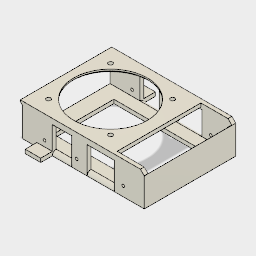
hard-drive-enclosure-v6 (Autodesk Fusion 360 design; units mm, degrees)
Autodesk Fusion 360 part; units mm, degrees
sketch "Sketch1" plane through (0, 0, 0) normal (0, 1, 0) x (1, 0, 0)
  line L0 (68.6494, -55) -> (-78.3404, -55)
  line L1 (-78.3404, -55) -> (-78.3404, 53)
  line L2 (-78.3404, 53) -> (68.6494, 53)
  line L3 (68.6494, 53) -> (68.6494, -55)
  line L4 (78.6494, 58) -> (-78.6124, 58)
  line L5 (-78.6124, 58) -> (-78.6124, -60)
  line L6 (-78.6124, -60) -> (78.6494, -60)
  line L7 (78.6494, -60) -> (78.6494, 58)
  dimension "d1" = 146.9898
  dimension "d2" = 108
  dimension "d3" = 5
  dimension "d4" = 5
  dimension "d5" = 10
  measures "d1" distance of L1 L3
  measures "d2" distance of L0 L2
  measures "d3" distance of L2 L4
  measures "d4" distance of L0 L6
  measures "d5" distance of L3 L7
extrude "Extrude1" add sketch "Sketch1" along normal blind 5 contours L0 L1 L2 L3 | L4 L5 L6 L7
sketch "Sketch2" plane through (0, 5, 0) normal (0, 1, 0) x (-1, 0, 0)
  line L0 (-78.6494, 60) -> (-78.6494, -58)
  line L1 (-78.6494, -58) -> (78.6124, -58)
  line L2 (78.6124, -58) -> (78.6124, 60)
  line L3 (78.6124, 60) -> (-78.6494, 60)
  line L4 (78.6124, -53) -> (-68.6494, -53)
  line L5 (-68.6494, -53) -> (-68.6494, 55)
  line L6 (-68.6494, 55) -> (78.6124, 55)
  line L7 (78.6124, 55) -> (78.6124, -53)
  line L8 (78.6124, -58) -> (-78.6494, -58)
  line L9 (-78.6494, -58) -> (-78.6494, 60)
  line L10 (-78.6494, 60) -> (78.6124, 60)
  line L11 (78.6124, 60) -> (78.6124, -58)
  dimension "d8" = 5
  dimension "d9" = 5
  dimension "d10" = 10
  measures "d8" distance of L1 L4
  measures "d9" distance of L3 L6
  measures "d10" distance of L0 L5
extrude "Extrude2" add sketch "Sketch2" along normal blind 27 contours L0 L1 L2 L3 L4 L5 L6 L8 L9 L10 L11
sketch "Sketch3" plane through (0, 32, 0) normal (0, 1, 0) x (-1, 0, 0)
  line L0 (78.6124, -53) -> (-68.6494, -53)
  line L1 (-68.6494, -53) -> (-68.6494, 55)
  line L2 (-68.6494, 55) -> (78.6124, 55)
  line L3 (78.6124, 55) -> (78.6124, 60)
  line L4 (78.6124, 60) -> (-78.6494, 60)
  line L5 (-78.6494, 60) -> (-78.6494, -58)
  line L6 (-78.6494, -58) -> (78.6124, -58)
  line L7 (78.6124, -58) -> (78.6124, -53)
  line L8 (56.3506, -58) -> (26.3506, -58)
  line L9 (26.3506, -58) -> (26.3506, 60)
  line L10 (26.3506, 60) -> (56.3506, 60)
  line L11 (56.3506, 60) -> (56.3506, -58)
  line L12 (-43.6494, 60) -> (-13.6494, 60)
  line L13 (-13.6494, 60) -> (-13.6494, -58)
  line L14 (-13.6494, -58) -> (-43.6494, -58)
  line L15 (-43.6494, -58) -> (-43.6494, 60)
  dimension "d13" = 112
  dimension "d14" = 30
  dimension "d15" = 30
  dimension "d16" = 40
  dimension "d17" = 25
  measures "d14" distance of L13 L15
  measures "d15" distance of L9 L11
  measures "d16" distance of L9 L13
  measures "d17" distance of L1 L15
extrude "Extrude3" add sketch "Sketch3" along normal blind 5 contours L0 L6 L7 L11 | L0 L6 L8 L9 L11 | L0 L6 L9 L13 | L0 L2 L9 L13 | L2 L3 L4 L11 | L2 L4 L9 L10 L11 | L0 L6 L13 L14 L15 | L2 L4 L9 L13 | L0 L1 L2 L4 L5 L6 L15 | L2 L4 L12 L13 L15
sketch "Sketch4" plane through (0, 0, 0) normal (0, -1, 0) x (1, 0, 0)
  line L0 (78.6494, -58) -> (78.6494, 60)
  line L1 (78.6494, 60) -> (-78.6124, 60)
  line L2 (-78.6124, 60) -> (-78.6124, -58)
  line L3 (-78.6124, -58) -> (78.6494, -58)
  line L4 (-60, 75) -> (-40, 75)
  line L5 (-40, 75) -> (-40, -73)
  line L6 (-40, -73) -> (-60, -73)
  line L7 (-60, -73) -> (-60, 75)
  line L8 (50, -73) -> (30, -73)
  line L9 (30, -73) -> (30, 75)
  line L10 (30, 75) -> (50, 75)
  line L11 (50, 75) -> (50, -73)
  dimension "d20" = 15
  dimension "d21" = 15
  dimension "d22" = 15
  dimension "d23" = 15
  measures "d20" distance of L1 L10
  measures "d21" distance of L3 L8
  measures "d22" distance of L3 L6
  measures "d23" distance of L1 L4
extrude "Extrude4" add sketch "Sketch4" against normal blind 5 contours L3 L8 L9 L11 | L1 L9 L10 L11 | L3 L5 L6 L7 | L1 L4 L5 L7
sketch "Sketch5" plane through (0, 0, 60) normal (0, 0, 1) x (1, 0, 0)
  line L0 (50, 5) -> (50, 0)
  line L1 (50, 0) -> (78.6494, 0)
  line L2 (78.6494, 0) -> (78.6494, 37)
  line L3 (78.6494, 37) -> (-78.6124, 37)
  line L4 (-78.6124, 37) -> (-78.6124, 0)
  line L5 (-78.6124, 0) -> (-60, 0)
  line L6 (-60, 0) -> (-60, 5)
  line L7 (-60, 5) -> (-40, 5)
  line L8 (-40, 5) -> (-40, 0)
  line L9 (-40, 0) -> (30, 0)
  line L10 (30, 0) -> (30, 5)
  line L11 (30, 5) -> (50, 5)
  circle A0 centre (-50.1136, 12.35) radius 1.7525
  circle A1 centre (-8.5084, 12.35) radius 1.7525
  circle A2 centre (51.4864, 12.35) radius 1.7525
  dimension "d26" = 12.35
  dimension "d27" = 12.35
  dimension "d28" = 12.35
  dimension "d29" = 3.505
  dimension "d30" = 3.505
  dimension "d31" = 3.505
  dimension "d32" = 28.4988
  dimension "d33" = 41.6052
  dimension "d34" = 101.6
  measures "d26" distance of L1 A2.centre
  measures "d27" distance of L9 A1.centre
  measures "d28" distance of L9 A0.centre
  measures "d29" diameter of A2
  measures "d30" diameter of A1
  measures "d31" diameter of A0
  measures "d32" distance of L4 A0.centre
  measures "d33" distance of A0.centre A1.centre
  measures "d34" distance of A0.centre A2.centre
extrude "Extrude5" cut sketch "Sketch5" against normal blind 170 contours A0 | A1 | A2
delete_face "DeleteFace1" 1 faces at (43.3333, 5, 65)
delete_face "DeleteFace2" 1 faces at (43.3333, 5, -68)
sketch "Sketch6" plane through (0, 0, 0) normal (0, -1, 0) x (1, 0, 0)
  line L0 (-60, -58) -> (-60, -73)
  line L1 (-60, -73) -> (-40, -73)
  line L2 (-40, -73) -> (-40, -58)
  line L3 (-40, -58) -> (78.6494, -58)
  line L4 (78.6494, -58) -> (78.6494, 60)
  line L5 (78.6494, 60) -> (-40, 60)
  line L6 (-40, 60) -> (-40, 75)
  line L7 (-40, 75) -> (-60, 75)
  line L8 (-60, 75) -> (-60, 60)
  line L9 (-60, 60) -> (-78.6124, 60)
  line L10 (-78.6124, 60) -> (-78.6124, -58)
  line L11 (-78.6124, -58) -> (-60, -58)
  line L12 (-58.6124, 40) -> (58.6494, 40)
  line L13 (58.6494, 40) -> (58.6494, -38)
  line L14 (58.6494, -38) -> (-58.6124, -38)
  line L15 (-58.6124, -38) -> (-58.6124, 40)
  dimension "d37" = 20
  dimension "d38" = 20
  dimension "d39" = 20
  dimension "d40" = 20
  measures "d37" distance of L5 L12
  measures "d38" distance of L3 L14
  measures "d39" distance of L4 L13
  measures "d40" distance of L10 L15
extrude "Extrude6" cut sketch "Sketch6" against normal blind 10 contours L12 L13 L14 L15
sketch "Sketch7" plane through (0, 37, 0) normal (0, 1, 0) x (-1, 0, 0)
  line L0 (-13.6494, -53) -> (-68.6494, -53)
  line L1 (-68.6494, -53) -> (-68.6494, 55)
  line L2 (-68.6494, 55) -> (-13.6494, 55)
  line L3 (-13.6494, 55) -> (-13.6494, -53)
  line L4 (-78.6494, -58) -> (78.6124, -58)
  line L5 (78.6124, -58) -> (78.6124, -53)
  line L6 (78.6124, -53) -> (26.3506, -53)
  line L7 (26.3506, -53) -> (26.3506, 55)
  line L8 (26.3506, 55) -> (78.6124, 55)
  line L9 (78.6124, 55) -> (78.6124, 60)
  line L10 (78.6124, 60) -> (-78.6494, 60)
  line L11 (-78.6494, 60) -> (-78.6494, -58)
  line L12 (26.3506, -53) -> (-13.6494, -53)
  line L13 (-13.6494, -53) -> (-13.6494, 55)
  line L14 (-13.6494, 55) -> (26.3506, 55)
  line L15 (26.3506, 55) -> (26.3506, -53)
extrude "Extrude7" cut sketch "Sketch7" against normal blind 10 contours L3 L7 L12 L13 L14 L15
sketch "Sketch8" plane through (0, 37, 0) normal (0, 1, 0) x (-1, 0, 0)
  line L0 (78.6124, -53) -> (-68.6494, -53)
  line L1 (-68.6494, -53) -> (-68.6494, 55)
  line L2 (-68.6494, 55) -> (78.6124, 55)
  line L3 (78.6124, 55) -> (78.6124, 60)
  line L4 (78.6124, 60) -> (-78.6494, 60)
  line L5 (-78.6494, 60) -> (-78.6494, -58)
  line L6 (-78.6494, -58) -> (78.6124, -58)
  line L7 (78.6124, -58) -> (78.6124, -53)
  line L8 (81.3506, -58) -> (-38.6494, -58)
  line L9 (-38.6494, -58) -> (-38.6494, 60)
  line L10 (-38.6494, 60) -> (81.3506, 60)
  line L11 (81.3506, 60) -> (81.3506, -58)
  dimension "d45" = 120
  dimension "d46" = 30
  measures "d45" distance of L9 L11
  measures "d46" distance of L1 L9
extrude "Extrude8" add sketch "Sketch8" along normal blind 5 contours L0 L6 L7 L8 L9 | L0 L2 L3 L7 L8 L9 L10 L11 | L2 L3 L4 L9 L10
move_face "OffsetFaces1" offset 2 1 faces at (-39.5252, 37, 19)
sketch "Sketch9" plane through (0, 42, 0) normal (0, 1, 0) x (-1, 0, 0)
  line L0 (81.3506, 60) -> (-38.6494, 60)
  line L1 (-38.6494, 60) -> (-38.6494, -58)
  line L2 (-38.6494, -58) -> (81.3506, -58)
  line L3 (81.3506, -58) -> (81.3506, 60)
  line L4 (71.3506, -46.5) -> (-23.6494, -46.5)
  line L5 (-23.6494, -46.5) -> (-23.6494, 48.5)
  line L6 (-23.6494, 48.5) -> (71.3506, 48.5)
  line L7 (71.3506, 48.5) -> (71.3506, -46.5)
  circle A0 centre (23.8506, 1) radius 47.5
  circle A1 centre (63.8506, -39) radius 2.8
  line L8 (58.6124, -38) -> (58.6124, 40)
  line L9 (-58.6494, -38) -> (58.6124, -38)
  circle A2 centre (-16.1494, 41) radius 2.8
  circle A3 centre (63.8506, 41) radius 2.8
  circle A4 centre (-16.1494, -39) radius 2.8
  dimension "d50" = 95
  dimension "d51" = 95
  dimension "d52" = 11.5
  dimension "d53" = 8
  dimension "d54" = 15
  dimension "d55" = 2.5
  dimension "d56" = 5.6
  dimension "d57" = 5.6
  dimension "d58" = 5.6
  dimension "d60" = 7.5
  dimension "d61" = 7.5
  dimension "d64" = 7.5
  dimension "d65" = 7.5
  dimension "d66" = 7.5
  dimension "d67" = 7.5
  dimension "d79" = 2.5
  dimension "d81" = 5.6
  dimension "d82" = 7.5
  dimension "d83" = 7.5
  measures "d50" distance of L5 L7
  measures "d51" distance of L4 L6
  measures "d52" distance of L0 L6
  measures "d54" distance of L1 L5
  measures "d56" diameter of A3
  measures "d57" diameter of A1
  measures "d58" diameter of A2
  measures "d60" distance of L4 A1.centre
  measures "d61" distance of L7 A1.centre
  measures "d64" distance of L5 A2.centre
  measures "d65" distance of L6 A2.centre
  measures "d66" distance of L6 A3.centre
  measures "d67" distance of L7 A3.centre
  measures "d81" diameter of A4
  measures "d82" distance of L5 A4.centre
  measures "d83" distance of L4 A4.centre
extrude "Extrude9" cut sketch "Sketch9" against normal blind 20 contours A0 L9 | A0 L8 | A0 L8 L9 | L9 A4 | L9 A4 | A1 | A2 | A3 picked at (37.1903, -12.7965)
sketch "Sketch10" plane through (0, 0, 60) normal (0, 0, 1) x (1, 0, 0)
  circle A0 centre (51.4864, 12.35) radius 1.7525
  circle A1 centre (-8.5084, 12.35) radius 1.7525
  circle A2 centre (-50.1136, 12.35) radius 1.7525
  line L0 (-78.6124, 35) -> (-78.6124, 0)
  line L1 (-78.6124, 0) -> (-60, 0)
  line L2 (-60, 0) -> (-60, 5)
  line L3 (-60, 5) -> (-40, 5)
  line L4 (-40, 5) -> (-40, 0)
  line L5 (-40, 0) -> (78.6494, 0)
  line L6 (78.6494, 0) -> (78.6494, 37)
  line L7 (78.6494, 37) -> (38.6494, 37)
  line L8 (38.6494, 37) -> (38.6494, 42)
  line L9 (38.6494, 42) -> (-81.3506, 42)
  line L10 (-81.3506, 42) -> (-81.3506, 35)
  line L11 (-81.3506, 35) -> (-78.6124, 35)
  line L12 (-40, 0) -> (-15, 0)
  line L13 (-15, 0) -> (-15, 35)
  line L14 (-15, 35) -> (-40, 35)
  line L15 (-40, 35) -> (-40, 0)
  line L16 (-78.6124, 35) -> (38.6494, 35)
  line L17 (5, 35) -> (40, 35)
  line L18 (40, 35) -> (40, 5)
  line L19 (40, 5) -> (5, 5)
  line L20 (5, 5) -> (5, 35)
  line L21 (-40, 35) -> (-15, 35)
  line L22 (-15, 35) -> (-15, 5)
  line L23 (-15, 5) -> (-40, 5)
  line L24 (-40, 5) -> (-40, 35)
  dimension "d70" = 25
  dimension "d71" = 35
  dimension "d72" = 30
  dimension "d73" = 20
  dimension "d76" = 35
  measures "d70" distance of L13 L15
  measures "d71" distance of L18 L20
  measures "d72" distance of L17.start L19.end
  measures "d73" distance of L13 L20
  measures "d76" distance of L12 L14
extrude "Extrude11" cut sketch "Sketch10" against normal blind 175 contours L13 L14 L15 L16 L21 L22 L23 L24 | L16 L17 L18 L19 L20
sketch "Sketch11" plane through (0, 0, 0) normal (0, -1, 0) x (1, 0, 0)
  line L0 (58.6494, 40) -> (58.6494, -38)
  line L1 (58.6494, -38) -> (-58.6124, -38)
  line L2 (-58.6124, -38) -> (-58.6124, 40)
  line L3 (-58.6124, 40) -> (58.6494, 40)
  line L4 (-60, -58) -> (-60, -73)
  line L5 (-60, -73) -> (-40, -73)
  line L6 (-40, -73) -> (-40, -58)
  line L7 (-40, -58) -> (78.6494, -58)
  line L8 (78.6494, -58) -> (78.6494, 60)
  line L9 (78.6494, 60) -> (-40, 60)
  line L10 (-40, 60) -> (-40, 75)
  line L11 (-40, 75) -> (-60, 75)
  line L12 (-60, 75) -> (-60, 60)
  line L13 (-60, 60) -> (-78.6124, 60)
  line L14 (-78.6124, 60) -> (-78.6124, -58)
  line L15 (-78.6124, -58) -> (-60, -58)
chamfer "Chamfer1" distance 5 angle 45 1 edges at (20.4349, 35, -16.1767)
fillet "Fillet1" radius 22.5 1 edges at (68.6494, 37, 1)
fillet "Fillet2" radius 5 4 edges at (-27.5, 5, -58) (22.5, 5, -58) (22.5, 5, 60) (-27.5, 5, 60)
sketch "Sketch12" plane through (0, 37, 0) normal (0, 1, 0) x (-1, 0, 0)
  line L0 (-78.6494, 55) -> (-38.6494, 55)
  line L1 (-38.6494, 55) -> (-38.6494, 60)
  line L2 (-38.6494, 60) -> (-78.6494, 60)
  line L3 (-78.6494, 60) -> (-78.6494, 55)
  line L4 (-38.6494, 55) -> (-78.6494, 55)
  line L5 (-78.6494, 55) -> (-78.6494, 60)
  line L6 (-78.6494, 60) -> (-38.6494, 60)
  line L7 (-38.6494, 60) -> (-38.6494, 55)
  line L8 (-38.6494, -58) -> (-78.6494, -58)
  line L9 (-78.6494, -58) -> (-78.6494, -53)
  line L10 (-78.6494, -53) -> (-38.6494, -53)
  line L11 (-38.6494, -53) -> (-38.6494, -58)
  point P0 (-38.6494, -58)
  point P1 (-78.6494, -53)
extrude "Extrude12" add sketch "Sketch12" along normal blind 5
chamfer "Chamfer2" distance 5 angle 45 2 edges at (78.6494, 42, -55.5) (78.6494, 42, 57.5)
chamfer "Chamfer3" distance 5 angle 45 1 edges at (-81.3506, 35, 1)
sketch "Sketch13" plane through (-78.6124, 0, 0) normal (-1, 0, 0) x (0, 0, 1)
  line L0 (-58, 0) -> (60, 0)
  line L1 (60, 0) -> (60, 37.2618)
  line L2 (60, 37.2618) -> (55, 37.2618)
  line L3 (55, 37.2618) -> (55, 5)
  line L4 (55, 5) -> (-53, 5)
  line L5 (-53, 5) -> (-53, 37.2618)
  line L6 (-53, 37.2618) -> (-58, 37.2618)
  line L7 (-58, 37.2618) -> (-58, 0)
  line L8 (-53, 35) -> (55, 35)
  line L9 (55, 35) -> (55, 37.2618)
  line L10 (55, 37.2618) -> (-53, 37.2618)
  line L11 (-53, 37.2618) -> (-53, 35)
  point P0 (-53, 35)
extrude "Extrude13" cut sketch "Sketch13" against normal blind 125 contours L3 L5 L8 L9 L10 L11
equation "d4 = d3"
equation "d26 = 0.25 in + 6 mm"
equation "d27 = d26"
equation "d28 = d26"
equation "d30 = d29"
equation "d31 = d29"
equation "d57 = d56"
equation "d58 = d56"
equation "d61 = d60"
equation "d63 = d61"
equation "d64 = d63"
equation "d65 = d63"
equation "d66 = d61"
equation "d67 = d61"
equation "d81 = d56"
equation "d82 = d64"
equation "d83 = d61"
